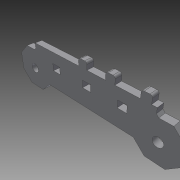
# Autodesk Inventor part: z_pulley_holder_left
Saved by Autodesk Inventor 2014 (Build 180170000, 170)
## iProperties
Created: 2014-04-03
Part Number: z_pulley_holder_left
Material: Plywood, Finish
Document SubType Name: Modeling
Designer: buben
Density: 0.552 g/cm^3
Appearance: Plywood - New
Author: buben
Autodesk Inventor part; units mm, degrees
ref_plane "YZ Plane" through (0, 0, 0) normal (1, 0, 0) x (0, 1, 0)
ref_plane "XZ Plane" through (0, 0, 0) normal (0, 1, 0) x (-1, 0, 0)
ref_plane "XY Plane" through (0, 0, 0) normal (0, 0, 1) x (1, 0, 0)
sketch "Sketch1" plane through (0, 0, 0) normal (0, 1, 0) x (-1, 0, 0)
  circle A0 centre (-18, -24.5) radius 13 construction
  circle A1 centre (-140.57, -24.5) radius 13 construction
  circle A2 centre (-4.1, -24.5) radius 0.9 construction
  circle A3 centre (-154.47, -24.5) radius 0.9 construction
  line L0 (0, -42.5) -> (-158.57, -42.5)
  line L1 (-158.57, -42.5) -> (-158.57, -6.5)
  line L2 (0, -6.5) -> (0, -42.5)
  line L3 (-22, -6.5) -> (-22, 0)
  line L4 (-22, 0) -> (-136.57, 0)
  line L5 (-136.57, 0) -> (-136.57, -6.5)
  line L6 (-158.57, -6.5) -> (-136.57, -6.5)
  line L7 (-22, -6.5) -> (0, -6.5)
  circle A4 centre (-18, -24.5) radius 17 construction
  circle A5 centre (-18, -24.5) radius 4.25
  circle A6 centre (-140.57, -24.5) radius 4.25
  point P0 (0, 0)
  point P1 (0, -24.5)
  dimension "d0" = 26
  dimension "d1" = 1.8
  dimension "d3" = 150.37
  dimension "d4" = 36
  dimension "d5" = 18
  dimension "d6" = 18
  dimension "d7" = 6.5
  dimension "d8" = 34
  dimension "d9" = 22
  dimension "d10" = 22
  dimension "d11" = 8.5
  constraints: 16 end point, 7 centre point, 5 horizontal alignment, 4 parallel, 4 perpendicular, 3 coincident, 3 equal radius, 2 tangent, 1 collinear, 1 horizontal, 1 midpoint, 1 vertical alignment
  measures "d0" diameter of A0
  measures "d1" diameter of A2
  measures "d3" distance of A3.centre A2.centre
  measures "d4" distance of L2.start L0.start
  measures "d5" distance from line of A0.centre L2
  measures "d6" distance from line of A1.centre L1
  measures "d7" distance of L4.end L5.end
  measures "d8" diameter of A4
  measures "d9" distance of L3.start L2.start
  measures "d10" distance of L1.end L5.end
  measures "d11" diameter of A5
extrude "Extrusion1" add sketch "Sketch1" along normal blind 6.5
chamfer "Chamfer1" distance 10 angle 45 4 edges at (0, 3.25, -42.5) (0, 3.25, -6.5) (158.57, 3.25, -6.5) (158.57, 3.25, -42.5)
sketch "Sketch2" plane through (0, 6.5, 0) normal (0, 1, 0) x (1, 0, 0)
  line L0 (148.57, 42.5) -> (10, 42.5) projected
  line L1 (158.57, 16.5) -> (148.57, 6.5) projected
  line L2 (158.57, 16.5) -> (158.57, 32.5) projected
  line L3 (26, 42.5) -> (36, 32.5)
  line L4 (36, 32.5) -> (122.57, 32.5)
  line L5 (122.57, 32.5) -> (132.57, 42.5)
  line L6 (26, 42.5) -> (132.57, 42.5)
  point P0 (0, 32.5)
  point P1 (0, 16.5)
  point P2 (0, 0)
  dimension "d17" = 10
  dimension "d18" = 16
  dimension "d19" = 16
  dimension "d20" = 16
  constraints: 8 end point, 3 perpendicular, 2 point on line, 1 collinear
  measures "d17" distance between parallel lines of L4 L6
  measures "d18" distance of point (0, 32.5) point (0, 16.5)
  measures "d19" distance of L3.start L0.end
  measures "d20" distance of L0.start L5.end
extrude "Extrusion2" cut sketch "Sketch2" against normal through all
sketch "Sketch3" plane through (0, 6.5, 0) normal (0, 1, 0) x (1, 0, 0)
  line L0 (22, 0) -> (136.57, 0) projected
  circle A0 centre (140.57, 24.5) radius 4.25 projected
  circle A1 centre (18, 24.5) radius 4.25 projected
  line L1 (36.57, 16.5) -> (121.57, 16.5) construction
  line L2 (121.57, 16.5) -> (121.57, 10) construction
  line L3 (121.57, 10) -> (36.57, 10) construction
  line L4 (36.57, 10) -> (36.57, 16.5) construction
  circle A2 centre (18, 24.5) radius 17 construction
  circle A3 centre (140.57, 24.5) radius 17 construction
  line L5 (42.57, 16.5) -> (50.57, 16.5)
  line L6 (50.57, 16.5) -> (50.57, 10)
  line L7 (50.57, 10) -> (42.57, 10)
  line L8 (42.57, 10) -> (42.57, 16.5)
  line L9 (75.07, 16.5) -> (83.07, 16.5)
  line L10 (83.07, 16.5) -> (83.07, 10)
  line L11 (83.07, 10) -> (75.07, 10)
  line L12 (75.07, 10) -> (75.07, 16.5)
  line L13 (107.57, 16.5) -> (115.57, 16.5)
  line L14 (115.57, 16.5) -> (115.57, 10)
  line L15 (115.57, 10) -> (107.57, 10)
  line L16 (107.57, 10) -> (107.57, 16.5)
  line L17 (50.57, 13.25) -> (75.07, 13.25) construction
  line L18 (83.07, 13.25) -> (107.57, 13.25) construction
  point P0 (0, 0)
  dimension "d23" = 6.5
  dimension "d24" = 85
  dimension "d25" = 34
  dimension "d26" = 34
  dimension "d27" = 19
  dimension "d28" = 10
  dimension "d29" = 8
  dimension "d30" = 6
  dimension "d31" = 6
  constraints: 36 end point, 8 parallel, 6 collinear, 4 horizontal, 4 midpoint, 4 perpendicular, 3 point on line, 2 centre point, 2 coincident
  measures "d23" distance of L3.end L1.start
  measures "d24" distance of L2.end L3.end
  measures "d25" diameter of A2
  measures "d26" diameter of A3
  measures "d27" distance from line of L2 A0.centre
  measures "d28" distance between parallel lines of L0 L3
  measures "d29" distance between parallel lines of L6 L8
  measures "d30" distance between parallel lines of L4 L8
  measures "d31" distance between parallel lines of L2 L14
extrude "Extrusion3" cut sketch "Sketch3" against normal through all contours L5 L6 L7 L8 | L9 L10 L11 L12 | L13 L14 L15 L16
chamfer "Chamfer2" distance 2 angle 45 2 edges at (22, 3.25, -6.5) (136.57, 3.25, -6.5)
sketch "Sketch4" plane through (0, 6.5, 0) normal (0, 1, 0) x (1, 0, 0)
  line L0 (22, 0) -> (136.57, 0) projected
  line L1 (136.57, 0) -> (136.57, 4.5) projected
  line L2 (132.57, 0) -> (124.57, 0)
  line L3 (124.57, 0) -> (124.57, -4.5)
  line L4 (126.57, -6.5) -> (130.57, -6.5)
  line L5 (132.57, -4.5) -> (132.57, 0)
  line L6 (104.57, 0) -> (96.57, 0)
  line L7 (96.57, 0) -> (96.57, -4.5)
  line L8 (98.57, -6.5) -> (102.57, -6.5)
  line L9 (104.57, -4.5) -> (104.57, 0)
  line L10 (79.57, 0) -> (71.57, 0)
  line L11 (71.57, 0) -> (71.57, -4.5)
  line L12 (73.57, -6.5) -> (77.57, -6.5)
  line L13 (79.57, -4.5) -> (79.57, 0)
  arc A0 (124.57, -4.5) -> (126.57, -6.5) centre (126.57, -4.5) ccw
  arc A1 (130.57, -6.5) -> (132.57, -4.5) centre (130.57, -4.5) ccw
  arc A2 (102.57, -6.5) -> (104.57, -4.5) centre (102.57, -4.5) ccw
  arc A3 (96.57, -4.5) -> (98.57, -6.5) centre (98.57, -4.5) ccw
  arc A4 (77.57, -6.5) -> (79.57, -4.5) centre (77.57, -4.5) ccw
  arc A5 (71.57, -4.5) -> (73.57, -6.5) centre (73.57, -4.5) ccw
  point P0 (0, 0)
  dimension "d37" = 2
  dimension "d38" = 8
  dimension "d39" = 8
  dimension "d40" = 8
  dimension "d41" = 6.5
  dimension "d42" = 4
  dimension "d43" = 20
  dimension "d44" = 45
  constraints: 24 end point, 12 point on circle, 12 tangent, 6 centre point, 6 parallel, 5 equal radius, 3 horizontal, 3 perpendicular, 3 point on line, 2 collinear
  measures "d37" radius of A0
  measures "d38" distance between parallel lines of L13 L11
  measures "d39" distance between parallel lines of L9 L7
  measures "d40" distance between parallel lines of L5 L3
  measures "d41" distance between parallel lines of L0 L4
  measures "d42" distance between parallel lines of L1 L5
  measures "d43" distance between parallel lines of L3 L9
  measures "d44" distance between parallel lines of L13 L3
extrude "Extrusion4" add sketch "Sketch4" against normal blind 6.5
equation "\"d5\" = 0.5 * d4"
equation "\"d6\" = d5"
equation "\"d10\" = d9"
equation "\"d19\" = d18"
equation "\"d20\" = d19"
equation "\"d31\" = d30"
equation "\"d39\" = d38"
equation "\"d40\" = d39"
body "Solid1"
